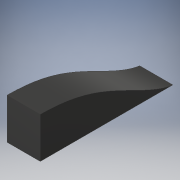
# Autodesk Inventor part: Ramp 1
Saved by Autodesk Inventor 2019 (Build 230136000, 136)
## iProperties
Created: 2020-04-28
Part Number: Ramp 1
Material: PBT Plastic
Document SubType Name: Modeling
Designer: infinity
Density: 1.31 g/cm^3
Appearance: Smooth - Black
Author: infinity
Autodesk Inventor part; units mm, degrees
ref_plane "YZ Plane" through (0, 0, 0) normal (1, 0, 0) x (0, 1, 0)
ref_plane "XZ Plane" through (0, 0, 0) normal (0, 1, 0) x (-1, 0, 0)
ref_plane "XY Plane" through (0, 0, 0) normal (0, 0, 1) x (1, 0, 0)
sketch "Sketch1" plane through (0, 0, 0) normal (1, 0, 0) x (0, 1, 0)
  line L0 (0, 0) -> (939.8, 0)
  line L1 (939.8, 0) -> (939.8, -3048)
  line L2 (939.8, -3048) -> (0, -3048)
  line L3 (0, -3048) -> (0, 0)
  spline S0 degree 4 poles (939.8, 0) (933.2373, -844.347) (775.2602, -1597.5655) (104.9883, -2340.5757) (0, -3048) knots 0 0 0 0 0 1 1 1 1 1
  point P0 (856.3439, -829.8243)
  point P1 (599.6038, -1607.5959)
  point P2 (237.1471, -2366.4895)
  dimension "d0" = 939.8
  dimension "d1" = 3048
  constraints: 8 end point, 2 parallel, 1 horizontal, 1 perpendicular, 5 other
  measures "d0" distance of L0.start L0.end
  measures "d1" distance of L2.end L0.start
extrude "Extrusion1" add sketch "Sketch1" along normal blind 762 contours L0 S0 L3
shell "Shell1" thickness 25.4 removed faces 1 at (508, 0, -1016)
body "Solid1"
